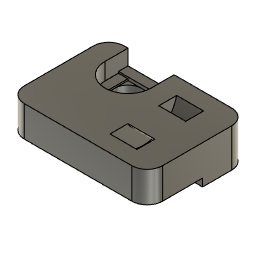
2020 Zip Tie Mount Asymmetric v2 (Autodesk Fusion 360 design; units mm, degrees)
Autodesk Fusion 360 part; units mm, degrees
note: some values were not read from the file. Set by a fixed rule: which sketch regions a step uses.
sketch "Sketch1" plane through (0, 0, 0) normal (0, 0, 1) x (1, 0, 0)
  line L0 (9, 3) -> (-9, 3)
  line L1 (-9, 3) -> (-9, -10)
  line L2 (-9, -10) -> (9, -10)
  line L3 (9, -10) -> (9, 3)
  circle A0 centre (-3.5, 0) radius 1.75
  circle A1 centre (-3.5, 0) radius 3
  line L4 (9, -2.8) -> (-9, -2.8)
  line L5 (-9, -2.8) -> (-9, 2.8)
  line L6 (-9, 2.8) -> (9, 2.8)
  line L7 (9, 2.8) -> (9, -2.8)
  line L8 (9, -2.8) -> (-9, 2.8) construction
  line L9 (-9, -2.8) -> (9, 2.8) construction
  dimension "d1" = 18
  dimension "d2" = 13
  dimension "d5" = 3.5
  dimension "d6" = 6
  dimension "d9" = 5.6
  dimension "d12" = 3.5
  dimension "d23" = 3
  constraint horizontal L0
  constraint perpendicular L0 L1
  constraint parallel L0 L2
  constraint parallel L1 L3
  constraint concentric A0 A1
  constraint horizontal L4
  constraint perpendicular L4 L5
  constraint parallel L4 L6
  constraint parallel L5 L7
  constraint coincident L3 L4.start
  constraint coincident L8 origin
  constraint coincident L9 origin
  constraint horizontal origin A0.centre
  measures "d1" distance of L1.end L2.end
  measures "d2" distance of L0.end L1.end
  measures "d5" diameter of A0
  measures "d6" diameter of A1
  measures "d9" distance of L4 L6
  measures "d12" distance of origin A0.centre
  measures "d23" distance of L0 A0.centre
extrude "Extrude1" add sketch "Sketch1" along normal blind 2
extrude "Extrude2" add sketch "Sketch1" along normal blind 4 contours L0 L3 A1 L6 | L0 L1 A1 L6 | L3 A1 L4 L6 L7 | L1 A1 L4 L5 L6 | L1 L2 L3 A1 L4
extrude "Extrude3" add sketch "Sketch1" against normal blind 1 contours L3 A1 L4 L6 L7 | A1 L4 L6 | L1 A1 L4 L5 L6
sketch "Sketch2" plane through (9, 0, 0) normal (1, 0, 0) x (0, 1, 0)
  line L0 (-10, 0) -> (-2.8, 0)
  line L1 (-2.8, 0) -> (-2.8, -1)
  line L2 (-2.8, -1) -> (2.8, -1)
  line L3 (2.8, -1) -> (2.8, 0)
  line L4 (2.8, 0) -> (3, 0)
  line L5 (3, 0) -> (3, 4)
  line L6 (3, 4) -> (-10, 4)
  line L7 (-10, 4) -> (-10, 0)
  circle A0 centre (-3.5, 5) radius 2.25
  circle A1 centre (-3.5, 5) radius 4.45
  line L8 (-10, 0) -> (3, 0)
  line L9 (-3.5, 4) -> (-3.5, 5) construction
  dimension "d13" = 4.5
  dimension "d14" = 2.2
  dimension "d18" = 5
  constraint concentric A0 A1
  constraint midpoint L6 L9.start
  constraint perpendicular L6 L9
  constraint coincident A0.centre A1.centre
  measures "d13" diameter of A0
  measures "d14" distance of A0 A1
  measures "d18" distance of A0.centre L8
extrude "Extrude4" cut sketch "Sketch2" against normal blind 3.5 from surface at -3.5 contours L6 A0 A1 picked at (-3.7762, 1.3019)
sketch "Sketch3" plane through (0, 0, 4) normal (0, 0, 1) x (-1, 0, 0)
  line L0 (-2, 5.5156) -> (-5.5, 5.5156)
  line L1 (-5.5, 5.5156) -> (-5.5, 7.8362)
  line L2 (-5.5, 7.8362) -> (-2, 7.8362)
  line L3 (-2, 7.8362) -> (-2, 5.5156)
  line L4 (-5.5, 1.4844) -> (-2, 1.4844)
  line L5 (-2, 1.4844) -> (-2, -0.8362)
  line L6 (-2, -0.8362) -> (-5.5, -0.8362)
  line L7 (-5.5, -0.8362) -> (-5.5, 1.4844)
  line L8 (-9, 10) -> (-9, -3)
  line L9 (-9, -3) -> (3.5, -3)
  circle A0 centre (3.5, 0) radius 3
  line L10 (3.5, -3) -> (9, -3)
  line L11 (9, -3) -> (9, 10)
  line L12 (9, 10) -> (-9, 10)
  line L13 (0.5, 0) -> (0.5, -5.3952)
  arc A1 (0.5, -5.3952) -> (6.5, -5.3952) centre (3.5, -5.3952) ccw
  line L14 (6.5, -5.3952) -> (6.5, 0)
  arc A2 (6.5, 0) -> (0.5, 0) centre (3.5, 0) ccw
  line L15 (3.5, 0) -> (3.5, -5.3952) construction
  constraint tangent L13 A1
  constraint tangent A1 L14
  constraint parallel L13 L14
  constraint tangent L14 A2
  constraint tangent L13 A2
  constraint perpendicular L10 L15
  constraint coincident A0.centre A2.centre
  constraint equal A0 A2
extrude "Extrude5" cut sketch "Sketch3" against normal up to surface (2 mm away) contours L9 A0 L13 | A0 L10 L14
fillet "Fillet1" radius 2 4 edges at (-9, -10, 2) (9, -10, 2) (9, 3, 2) (-9, 3, 2)
sketch "Sketch4" plane through (0, 0, 2) normal (0, 0, 1) x (-1, 0, 0)
  arc A0 (6.5, 0) -> (0.5, 0) centre (3.5, 0) ccw
  line L0 (0.5, 0) -> (0.5, -3)
  line L1 (0.5, -3) -> (6.5, -3)
  line L2 (6.5, -3) -> (6.5, 0)
  circle A1 centre (3.5, 0) radius 1.75 construction
  line L3 (0.5, -1.75) -> (6.5, -1.75)
  line L4 (5.25, -1.75) -> (5.25, 1.75)
  line L5 (5.9367, 1.75) -> (1.0633, 1.75)
  line L6 (1.75, 1.75) -> (1.75, -1.75)
  line L7 (1.75, -1.75) -> (5.25, 1.75) construction
  line L8 (5.25, -1.75) -> (1.75, 1.75) construction
  point P0 (3.5, 0)
  constraint horizontal L3
  constraint perpendicular L3 L4
  constraint parallel L3 L5
  constraint parallel L4 L6
  constraint coincident L7 P0
  constraint coincident L8 P0
  constraint coincident P0 A0.centre
  constraint tangent A1 L3
  constraint tangent A1 L6
  constraint coincident L2 L3.end
  constraint coincident L4.start L3
  constraint coincident A0 L5.start
  constraint coincident L4.end L5
  constraint coincident A0 L5.end
  constraint coincident L6.start L5
  constraint coincident L0 L3.start
  constraint coincident L6.end L3
extrude "Extrude6" cut sketch "Sketch4" against normal blind 0.2 contours A0 L2 L3 L4 L5 | A0 L0 L3 L5 L6 | L3 L4 L5 L6
extrude "Extrude7" cut sketch "Sketch4" against normal blind 0.4 contours L3 L4 L5 L6
